Autodesk Fusion 360 part; units mm, degrees
(part 4 of 4)
  spline S3 degree 5 poles (40.8877, 43.7518) (40.9094, 43.7499) (40.9529, 43.7455) (41.018, 43.7374) (41.1043, 43.7233) (41.2113, 43.6998) (41.317, 43.6706) (41.4211, 43.6359) (41.5232, 43.5957) (41.6229, 43.5502) (41.7199, 43.4994) (41.8136, 43.4432) (41.9039, 43.3818) (41.9906, 43.3154) (42.0736, 43.2441) (42.1528, 43.1684) (42.2283, 43.0887) (42.3, 43.0054) (42.3678, 42.9189) (42.4312, 42.8292) (42.4898, 42.7365) (42.5431, 42.641) (42.5907, 42.5425) (42.6323, 42.4415) (42.6679, 42.338) (42.6976, 42.2325) (42.7216, 42.1254) (42.7401, 42.0171) (42.7532, 41.9082) (42.7608, 41.7988) (42.7627, 41.6893) (42.7587, 41.58) (42.7486, 41.4712) (42.7322, 41.3632) (42.7097, 41.2561) (42.6811, 41.1503) (42.6468, 41.0461) (42.6069, 40.9437) (42.5616, 40.8437) (42.511, 40.7464) (42.4551, 40.6523) (42.3941, 40.5617) (42.328, 40.475) (42.257, 40.3921) (42.1815, 40.3132) (42.1021, 40.238) (42.0191, 40.1663) (41.9329, 40.0981) (41.844, 40.0337) (41.7523, 39.9734) (41.6578, 39.9179) (41.5605, 39.8679) (41.4603, 39.8242) (41.3575, 39.787) (41.2523, 39.7567) (41.1453, 39.7331) (41.037, 39.7157) (40.9279, 39.704) (40.8186, 39.6971) (40.7091, 39.6938) (40.5997, 39.693) (40.4904, 39.6936) (40.381, 39.6947) (40.2717, 39.6955) (40.1623, 39.6958) (40.0529, 39.6956) (39.9435, 39.6951) (39.834, 39.6945) (39.7246, 39.6941) (39.6152, 39.694) (39.5058, 39.6941) (39.3964, 39.6944) (39.287, 39.6946) (39.1776, 39.6948) (39.0682, 39.6948) (38.9588, 39.6948) (38.8494, 39.6947) (38.74, 39.6946) (38.6306, 39.6945) (38.5212, 39.6945) (38.4118, 39.6945) (38.3024, 39.6945) (38.193, 39.6946) (38.0836, 39.6946) (37.9742, 39.6946) (37.8648, 39.6946) (37.7554, 39.6946) (37.646, 39.6946) (37.5366, 39.6946) (37.4272, 39.6946) (37.3178, 39.6946) (37.2084, 39.6946) (37.099, 39.6946) (36.9896, 39.6946) (36.8802, 39.6946) (36.7708, 39.6946) (36.6614, 39.6946) (36.552, 39.6946) (36.4425, 39.6946) (36.3331, 39.6946) (36.2237, 39.6946) (36.1143, 39.6946) (36.0049, 39.6946) (35.8955, 39.6946) (35.7861, 39.6946) (35.6767, 39.6946) (35.5673, 39.6946) (35.4579, 39.6946) (35.3485, 39.6945) (35.2391, 39.6945) (35.1297, 39.6945) (35.0203, 39.6945) (34.9109, 39.6946) (34.8015, 39.6946) (34.6922, 39.6947) (34.5828, 39.6947) (34.4734, 39.6947) (34.3639, 39.6946) (34.2544, 39.6944) (34.1449, 39.6943) (34.0355, 39.6942) (33.9262, 39.6943) (33.8169, 39.6946) (33.7077, 39.6949) (33.5984, 39.6952) (33.4891, 39.6952) (33.3796, 39.6949) (33.2699, 39.6945) (33.1601, 39.6949) (33.0503, 39.697) (32.9408, 39.7026) (32.832, 39.7131) (32.7241, 39.7298) (32.6176, 39.7538) (32.5128, 39.785) (32.41, 39.8233) (32.3094, 39.8679) (32.2115, 39.918) (32.1163, 39.9732) (32.0243, 40.033) (31.9357, 40.0972) (31.8507, 40.1659) (31.7695, 40.239) (31.6923, 40.3165) (31.6193, 40.3982) (31.5506, 40.4837) (31.4863, 40.5727) (31.4266, 40.6647) (31.3715, 40.7596) (31.3215, 40.8569) (31.2765, 40.9566) (31.237, 41.0585) (31.203, 41.1625) (31.1748, 41.2682) (31.1527, 41.3755) (31.1366, 41.4839) (31.1266, 41.5931) (31.1229, 41.7026) (31.1253, 41.8121) (31.1336, 41.9212) (31.1477, 42.0297) (31.1675, 42.1374) (31.1927, 42.244) (31.2232, 42.3492) (31.2592, 42.4526) (31.3007, 42.5538) (31.3478, 42.6525) (31.4006, 42.7483) (31.459, 42.8409) (31.5226, 42.93) (31.5911, 43.0155) (31.6642, 43.0974) (31.7412, 43.1754) (31.822, 43.2495) (31.9062, 43.3196) (31.9937, 43.3855) (32.0844, 43.447) (32.1781, 43.5038) (32.2748, 43.5555) (32.3743, 43.6017) (32.4762, 43.6419) (32.5802, 43.6759) (32.686, 43.7035) (32.7933, 43.7249) (32.9016, 43.7405) (33.0106, 43.7511) (33.1201, 43.7577) (33.2297, 43.7613) (33.3393, 43.7627) (33.4487, 43.7627) (33.5581, 43.7621) (33.6674, 43.7612) (33.7767, 43.7605) (33.886, 43.76) (33.9954, 43.7599) (34.1048, 43.76) (34.2142, 43.7603) (34.3237, 43.7606) (34.4331, 43.7608) (34.5426, 43.7609) (34.6519, 43.7608) (34.7613, 43.7607) (34.8707, 43.7606) (34.9801, 43.7605) (35.0895, 43.7605) (35.1989, 43.7605) (35.3083, 43.7605) (35.4177, 43.7606) (35.5271, 43.7606) (35.6365, 43.7606) (35.7459, 43.7606) (35.8553, 43.7606) (35.9647, 43.7606) (36.0741, 43.7606) (36.1835, 43.7606) (36.2929, 43.7606) (36.4023, 43.7606) (36.5117, 43.7606) (36.6211, 43.7606) (36.7305, 43.7606) (36.84, 43.7606) (36.9494, 43.7606) (37.0588, 43.7606) (37.1682, 43.7606) (37.2776, 43.7606) (37.387, 43.7606) (37.4964, 43.7606) (37.6058, 43.7606) (37.7152, 43.7606) (37.8246, 43.7605) (37.934, 43.7605) (38.0434, 43.7605) (38.1528, 43.7606) (38.2622, 43.7606) (38.3716, 43.7607) (38.481, 43.7607) (38.5904, 43.7607) (38.6998, 43.7606) (38.8092, 43.7604) (38.9186, 43.7603) (39.028, 43.7602) (39.1374, 43.7603) (39.2468, 43.7606) (39.3562, 43.7609) (39.4656, 43.7612) (39.5751, 43.7613) (39.6844, 43.7612) (39.7938, 43.7606) (39.9032, 43.7598) (40.0125, 43.7591) (40.1219, 43.7588) (40.2313, 43.7593) (40.3408, 43.7605) (40.4503, 43.7621) (40.5599, 43.7635) (40.6694, 43.7632) (40.7568, 43.7608) (40.8223, 43.7571) (40.8659, 43.7538) (40.8877, 43.7518) knots 0 0 0 0 0 0 0.00392157 0.00784314 0.01176471 0.01568627 0.01960784 0.02352941 0.02745098 0.03137255 0.03529412 0.03921569 0.04313725 0.04705882 0.05098039 0.05490196 0.05882353 0.0627451 0.06666667 0.07058824 0.0745098 0.07843137 0.08235294 0.08627451 0.09019608 0.09411765 0.09803922 0.10196078 0.10588235 0.10980392 0.11372549 0.11764706 0.12156863 0.1254902 0.12941176 0.13333333 0.1372549 0.14117647 0.14509804 0.14901961 0.15294118 0.15686275 0.16078431 0.16470588 0.16862745 0.17254902 0.17647059 0.18039216 0.18431373 0.18823529 0.19215686 0.19607843 0.2 0.20392157 0.20784314 0.21176471 0.21568627 0.21960784 0.22352941 0.22745098 0.23137255 0.23529412 0.23921569 0.24313725 0.24705882 0.25098039 0.25490196 0.25882353 0.2627451 0.26666667 0.27058824 0.2745098 0.27843137 0.28235294 0.28627451 0.29019608 0.29411765 0.29803922 0.30196078 0.30588235 0.30980392 0.31372549 0.31764706 0.32156863 0.3254902 0.32941176 0.33333333 0.3372549 0.34117647 0.34509804 0.34901961 0.35294118 0.35686275 0.36078431 0.36470588 0.36862745 0.37254902 0.37647059 0.38039216 0.38431373 0.38823529 0.39215686 0.39607843 0.4 0.40392157 0.40784314 0.41176471 0.41568627 0.41960784 0.42352941 0.42745098 0.43137255 0.43529412 0.43921569 0.44313725 0.44705882 0.45098039 0.45490196 0.45882353 0.4627451 0.46666667 0.47058824 0.4745098 0.47843137 0.48235294 0.48627451 0.49019608 0.49411765 0.49803922 0.50196078 0.50588235 0.50980392 0.51372549 0.51764706 0.52156863 0.5254902 0.52941176 0.53333333 0.5372549 0.54117647 0.54509804 0.54901961 0.55294118 0.55686275 0.56078431 0.56470588 0.56862745 0.57254902 0.57647059 0.58039216 0.58431373 0.58823529 0.59215686 0.59607843 0.6 0.60392157 0.60784314 0.61176471 0.61568627 0.61960784 0.62352941 0.62745098 0.63137255 0.63529412 0.63921569 0.64313725 0.64705882 0.65098039 0.65490196 0.65882353 0.6627451 0.66666667 0.67058824 0.6745098 0.67843137 0.68235294 0.68627451 0.69019608 0.69411765 0.69803922 0.70196078 0.70588235 0.70980392 0.71372549 0.71764706 0.72156863 0.7254902 0.72941176 0.73333333 0.7372549 0.74117647 0.74509804 0.74901961 0.75294118 0.75686275 0.76078431 0.76470588 0.76862745 0.77254902 0.77647059 0.78039216 0.78431373 0.78823529 0.79215686 0.79607843 0.8 0.80392157 0.80784314 0.81176471 0.81568627 0.81960784 0.82352941 0.82745098 0.83137255 0.83529412 0.83921569 0.84313725 0.84705882 0.85098039 0.85490196 0.85882353 0.8627451 0.86666667 0.87058824 0.8745098 0.87843137 0.88235294 0.88627451 0.89019608 0.89411765 0.89803922 0.90196078 0.90588235 0.90980392 0.91372549 0.91764706 0.92156863 0.9254902 0.92941176 0.93333333 0.9372549 0.94117647 0.94509804 0.94901961 0.95294118 0.95686275 0.96078431 0.96470588 0.96862745 0.97254902 0.97647059 0.98039216 0.98431373 0.98823529 0.99215686 0.99607843 1 1 1 1 1 1
  point P0 (47.9215, 72.9576)
  point P1 (48.4702, 72.8769)
  point P2 (49.0161, 72.7805)
  point P3 (49.5581, 72.6648)
  point P4 (50.0918, 72.5165)
  point P5 (50.6215, 72.3558)
  point P6 (51.1435, 72.171)
  point P7 (51.6562, 71.9628)
  point P8 (52.1629, 71.7382)
  point P9 (52.6554, 71.4852)
  point P10 (53.1393, 71.215)
  point P11 (53.6132, 70.9281)
  point P12 (54.0761, 70.6237)
  point P13 (54.5279, 70.3027)
  point P14 (54.9671, 69.964)
  point P15 (55.3873, 69.6016)
  point P16 (55.7975, 69.2281)
  point P17 (56.1881, 68.834)
  point P18 (56.5593, 68.4216)
  point P19 (56.9182, 67.9986)
  point P20 (57.2575, 67.5599)
  point P21 (57.582, 67.1104)
  point P22 (57.8848, 66.6464)
  point P23 (58.1692, 66.171)
  point P24 (58.4379, 65.6865)
  point P25 (58.6841, 65.1896)
  point P26 (58.9068, 64.683)
  point P27 (59.1142, 64.1696)
  point P28 (59.5316, 63.8586)
  point P29 (60.0421, 63.6449)
  point P30 (60.5476, 63.4178)
  point P31 (61.042, 63.1672)
  point P32 (61.5236, 62.8936)
  point P33 (61.9946, 62.6021)
  point P34 (62.4534, 62.2913)
  point P35 (62.8966, 61.9579)
  point P36 (63.3303, 61.6119)
  point P37 (63.7474, 61.246)
  point P38 (64.1551, 60.8697)
  point P39 (64.5428, 60.4727)
  point P40 (64.9129, 60.0594)
  point P41 (65.2657, 59.6314)
  point P42 (65.6007, 59.1895)
  point P43 (65.9224, 58.738)
  point P44 (66.2228, 58.2724)
  point P45 (66.5057, 57.796)
  point P46 (66.7674, 57.3077)
  point P47 (67.0123, 56.8115)
  point P48 (67.2308, 56.3023)
  point P49 (67.4271, 55.7848)
  point P50 (67.606, 55.2606)
  point P51 (67.7736, 54.7327)
  point P52 (67.9053, 54.1944)
  point P53 (68.0248, 53.6533)
  point P54 (68.112, 53.1057)
  point P55 (68.1767, 52.5549)
  point P56 (68.2351, 52.0033)
  point P57 (68.249, 51.4486)
  point P58 (68.25, 50.8937)
  point P59 (68.2495, 50.3387)
  point P60 (68.2126, 49.7854)
  point P61 (68.1435, 49.235)
  point P62 (68.0572, 48.6872)
  point P63 (67.9523, 48.1428)
  point P64 (67.8163, 47.6059)
  point P65 (67.6733, 47.0707)
  point P66 (67.4992, 46.5447)
  point P67 (67.3027, 46.0271)
  point P68 (67.0815, 45.5197)
  point P69 (66.8456, 45.0184)
  point P70 (66.5847, 44.5296)
  point P71 (66.3047, 44.0517)
  point P72 (66.003, 43.5866)
  point P73 (65.683, 43.1338)
  point P74 (65.3446, 42.6943)
  point P75 (64.9949, 42.2641)
  point P76 (65.0476, 41.7178)
  point P77 (65.1148, 41.1677)
  point P78 (65.1637, 40.615)
  point P79 (65.1808, 40.0604)
  point P80 (65.1782, 39.5055)
  point P81 (65.1586, 38.9509)
  point P82 (65.1109, 38.3981)
  point P83 (65.0454, 37.8476)
  point P84 (64.9561, 37.3006)
  point P85 (64.8392, 36.759)
  point P86 (64.7059, 36.2212)
  point P87 (64.5429, 35.6918)
  point P88 (64.362, 35.1685)
  point P89 (64.1647, 34.6511)
  point P90 (63.9475, 34.1418)
  point P91 (63.7122, 33.6399)
  point P92 (63.4598, 33.1464)
  point P93 (63.1814, 32.6675)
  point P94 (62.8832, 32.2001)
  point P95 (62.5625, 31.7478)
  point P96 (62.2276, 31.3058)
  point P97 (61.8776, 30.8756)
  point P98 (61.5099, 30.4601)
  point P99 (61.1225, 30.0629)
  point P100 (60.7194, 29.6816)
  point P101 (60.3015, 29.3166)
  point P102 (59.869, 28.9693)
  point P103 (59.426, 28.636)
  point P104 (58.966, 28.3265)
  point P105 (58.4964, 28.0324)
  point P106 (58.0156, 27.7575)
  point P107 (57.5265, 27.4992)
  point P108 (57.0237, 27.2687)
  point P109 (56.5128, 27.0555)
  point P110 (55.9932, 26.8631)
  point P111 (55.4664, 26.6917)
  point P112 (54.9312, 26.5488)
  point P113 (54.3934, 26.4161)
  point P114 (53.8492, 26.3097)
  point P115 (53.3013, 26.2235)
  point P116 (52.749, 26.1699)
  point P117 (52.1966, 26.1203)
  point P118 (51.6418, 26.1074)
  point P119 (51.0869, 26.1104)
  point P120 (50.5323, 26.1285)
  point P121 (49.9803, 26.1839)
  point P122 (49.4297, 26.2488)
  point P123 (48.912, 26.1996)
  point P124 (48.4809, 25.8503)
  point P125 (48.0343, 25.5214)
  point P126 (47.5779, 25.2068)
  point P127 (47.1078, 24.9133)
  point P128 (46.6285, 24.636)
  point P129 (46.1351, 24.3838)
  point P130 (45.6315, 24.1538)
  point P131 (45.1199, 23.9423)
  point P132 (44.5994, 23.7539)
  point P133 (44.0704, 23.5904)
  point P134 (43.5373, 23.4403)
  point P135 (42.9951, 23.3256)
  point P136 (42.4494, 23.2296)
  point P137 (41.9007, 23.1492)
  point P138 (41.3496, 23.0854)
  point P139 (40.7955, 23.0575)
  point P140 (40.2406, 23.0536)
  point P141 (39.6857, 23.0563)
  point P142 (39.1314, 23.0801)
  point P143 (38.5804, 23.1453)
  point P144 (38.0317, 23.2253)
  point P145 (37.4859, 23.3214)
  point P146 (36.9434, 23.4345)
  point P147 (36.4092, 23.581)
  point P148 (35.8773, 23.7362)
  point P149 (35.3559, 23.9223)
  point P150 (34.8426, 24.13)
  point P151 (34.3375, 24.3561)
  point P152 (33.846, 24.6098)
  point P153 (33.3596, 24.8745)
  point P154 (32.8857, 25.1617)
  point P155 (32.4233, 25.4674)
  point P156 (31.9694, 25.7858)
  point P157 (31.5305, 26.1248)
  point P158 (31.1077, 26.4841)
  point P159 (30.6997, 26.8601)
  point P160 (30.3078, 27.253)
  point P161 (29.934, 27.663)
  point P162 (29.5741, 28.0853)
  point P163 (29.2332, 28.5228)
  point P164 (28.9115, 28.9744)
  point P165 (28.6046, 29.436)
  point P166 (28.3191, 29.9109)
  point P167 (28.0549, 30.3978)
  point P168 (27.8036, 30.8906)
  point P169 (27.5815, 31.3982)
  point P170 (27.3745, 31.9114)
  point P171 (26.9733, 32.2362)
  point P172 (26.4617, 32.4482)
  point P173 (25.9597, 32.6825)
  point P174 (25.4662, 32.9334)
  point P175 (24.9835, 33.2057)
  point P176 (24.5103, 33.4937)
  point P177 (24.0487, 33.8007)
  point P178 (23.6051, 34.1335)
  point P179 (23.1722, 34.4802)
  point P180 (22.7548, 34.8459)
  point P181 (22.3485, 35.2237)
  point P182 (21.9591, 35.619)
  point P183 (21.5898, 36.0332)
  point P184 (21.2339, 36.4586)
  point P185 (20.8999, 36.9012)
  point P186 (20.5778, 37.3526)
  point P187 (20.2804, 37.8205)
  point P188 (19.9966, 38.2963)
  point P189 (19.7306, 38.7817)
  point P190 (19.4885, 39.279)
  point P191 (19.2698, 39.7879)
  point P192 (19.0752, 40.306)
  point P193 (18.8954, 40.8301)
  point P194 (18.7319, 41.3593)
  point P195 (18.607, 41.8993)
  point P196 (18.4952, 42.442)
  point P197 (18.4017, 42.9883)
  point P198 (18.3273, 43.5376)
  point P199 (18.2664, 44.089)
  point P200 (18.2522, 44.6437)
  point P201 (18.2507, 45.1986)
  point P202 (18.263, 45.7533)
  point P203 (18.3192, 46.3051)
  point P204 (18.3818, 46.8562)
  point P205 (18.4663, 47.4043)
  point P206 (18.5782, 47.9472)
  point P207 (18.7076, 48.4859)
  point P208 (18.8631, 49.0172)
  point P209 (19.0348, 49.5435)
  point P210 (19.2319, 50.0607)
  point P211 (19.4442, 50.572)
  point P212 (19.6738, 51.0764)
  point P213 (19.9353, 51.5652)
  point P214 (20.2124, 52.0448)
  point P215 (20.507, 52.5143)
  point P216 (20.8178, 52.9729)
  point P217 (21.1502, 53.4169)
  point P218 (21.4924, 53.8519)
  point P219 (21.422, 54.3987)
  point P220 (21.3645, 54.9506)
  point P221 (21.3157, 55.503)
  point P222 (21.3041, 56.0578)
  point P223 (21.3057, 56.6127)
  point P224 (21.3199, 57.1674)
  point P225 (21.3719, 57.7197)
  point P226 (21.4294, 58.2715)
  point P227 (21.5206, 58.8185)
  point P228 (21.6429, 59.359)
  point P229 (21.7782, 59.8963)
  point P230 (21.9446, 60.4246)
  point P231 (22.1245, 60.9482)
  point P232 (22.3222, 61.4655)
  point P233 (22.5361, 61.9763)
  point P234 (22.7746, 62.4755)
  point P235 (23.0264, 62.9679)
  point P236 (23.3058, 63.4464)
  point P237 (23.6041, 63.9133)
  point P238 (23.9246, 64.3658)
  point P239 (24.2582, 64.8088)
  point P240 (24.6097, 65.2377)
  point P241 (24.9763, 65.6542)
  point P242 (25.3623, 66.0528)
  point P243 (25.7624, 66.4373)
  point P244 (26.1835, 66.7984)
  point P245 (26.6196, 67.1408)
  point P246 (27.0633, 67.4732)
  point P247 (27.5223, 67.7838)
  point P248 (27.9918, 68.0779)
  point P249 (28.4735, 68.3509)
  point P250 (28.9625, 68.6097)
  point P251 (29.4659, 68.8387)
  point P252 (29.9766, 69.0525)
  point P253 (30.4964, 69.2442)
  point P254 (31.0235, 69.415)
  point P255 (31.5587, 69.5575)
  point P256 (32.0967, 69.6893)
  point P257 (32.6408, 69.7961)
  point P258 (33.1891, 69.8796)
  point P259 (33.7414, 69.9332)
  point P260 (34.2938, 69.9843)
  point P261 (34.8485, 69.9981)
  point P262 (35.4034, 69.9954)
  point P263 (35.9578, 69.9741)
  point P264 (36.51, 69.9199)
  point P265 (37.0599, 69.8501)
  point P266 (37.577, 69.9106)
  point P267 (38.0109, 70.2562)
  point P268 (38.4612, 70.5799)
  point P269 (38.9196, 70.8915)
  point P270 (39.3913, 71.182)
  point P271 (39.8744, 71.4536)
  point P272 (40.3698, 71.7007)
  point P273 (40.8725, 71.9333)
  point P274 (41.3859, 72.1404)
  point P275 (41.9068, 72.3273)
  point P276 (42.4336, 72.4984)
  point P277 (42.968, 72.6441)
  point P278 (43.5077, 72.7697)
  point P279 (44.0531, 72.869)
  point P280 (44.6016, 72.951)
  point P281 (45.1534, 73.0092)
  point P282 (45.7065, 73.049)
  point P283 (46.2614, 73.0553)
  point P284 (46.8163, 73.0505)
  point P285 (47.2756, 68.9919)
  point P286 (47.8251, 68.9156)
  point P287 (48.3701, 68.8132)
  point P288 (48.9103, 68.6871)
  point P289 (49.4398, 68.523)
  point P290 (49.961, 68.3348)
  point P291 (50.4679, 68.1112)
  point P292 (50.9607, 67.8585)
  point P293 (51.4374, 67.5749)
  point P294 (51.8924, 67.2574)
  point P295 (52.3321, 66.9186)
  point P296 (52.756, 66.5601)
  point P297 (53.1568, 66.1755)
  point P298 (53.5396, 65.773)
  point P299 (53.8939, 65.3456)
  point P300 (54.2267, 64.9014)
  point P301 (54.5295, 64.4364)
  point P302 (54.8078, 63.957)
  point P303 (55.0547, 63.4603)
  point P304 (55.2788, 62.9538)
  point P305 (55.4736, 62.4346)
  point P306 (55.6467, 61.908)
  point P307 (55.8439, 61.3916)
  point P308 (56.1684, 60.9439)
  point P309 (56.6144, 60.6169)
  point P310 (57.1298, 60.4154)
  point P311 (57.6624, 60.2612)
  point P312 (58.1825, 60.0688)
  point P313 (58.6887, 59.8441)
  point P314 (59.1863, 59.5983)
  point P315 (59.6702, 59.3281)
  point P316 (60.1341, 59.024)
  point P317 (60.5823, 58.697)
  point P318 (61.0061, 58.3382)
  point P319 (61.4132, 57.9604)
  point P320 (61.7929, 57.5552)
  point P321 (62.1547, 57.1339)
  point P322 (62.4843, 56.6872)
  point P323 (62.7899, 56.2241)
  point P324 (63.0633, 55.7416)
  point P325 (63.3145, 55.2481)
  point P326 (63.535, 54.7393)
  point P327 (63.7263, 54.2194)
  point P328 (63.893, 53.6906)
  point P329 (64.0167, 53.1498)
  point P330 (64.1187, 52.6046)
  point P331 (64.1905, 52.0545)
  point P332 (64.2385, 51.5012)
  point P333 (64.2479, 50.9458)
  point P334 (64.2119, 50.3917)
  point P335 (64.163, 49.8384)
  point P336 (64.0742, 49.2904)
  point P337 (63.9592, 48.7474)
  point P338 (63.8113, 48.213)
  point P339 (63.6315, 47.689)
  point P340 (63.4266, 47.174)
  point P341 (63.1862, 46.6738)
  point P342 (62.9229, 46.1855)
  point P343 (62.6334, 45.7126)
  point P344 (62.3179, 45.256)
  point P345 (61.971, 44.8224)
  point P346 (61.5993, 44.4098)
  point P347 (61.2232, 44.0018)
  point P348 (60.9522, 43.52)
  point P349 (60.8425, 42.9787)
  point P350 (60.8875, 42.4271)
  point P351 (61.0221, 41.8889)
  point P352 (61.1234, 41.3433)
  point P353 (61.2017, 40.7936)
  point P354 (61.2354, 40.2392)
  point P355 (61.2458, 39.6839)
  point P356 (61.2258, 39.1288)
  point P357 (61.1793, 38.5755)
  point P358 (61.0998, 38.0259)
  point P359 (60.9831, 37.4839)
  point P360 (60.8343, 36.9497)
  point P361 (60.6556, 36.4252)
  point P362 (60.4518, 35.9097)
  point P363 (60.2143, 35.4095)
  point P364 (59.9538, 34.9206)
  point P365 (59.664, 34.4475)
  point P366 (59.3438, 33.994)
  point P367 (58.9961, 33.5613)
  point P368 (58.6253, 33.1477)
  point P369 (58.2337, 32.7539)
  point P370 (57.8185, 32.385)
  point P371 (57.3815, 32.0427)
  point P372 (56.926, 31.7261)
  point P373 (56.4574, 31.4291)
  point P374 (55.9708, 31.1644)
  point P375 (55.4714, 30.9256)
  point P376 (54.9558, 30.7226)
  point P377 (54.4322, 30.5405)
  point P378 (53.9014, 30.3806)
  point P379 (53.3589, 30.2652)
  point P380 (52.8111, 30.1768)
  point P381 (52.2588, 30.1183)
  point P382 (51.7037, 30.1)
  point P383 (51.1483, 30.1068)
  point P384 (50.5948, 30.1498)
  point P385 (50.0438, 30.2173)
  point P386 (49.5028, 30.3389)
  point P387 (48.9638, 30.4682)
  point P388 (48.4135, 30.5203)
  point P389 (47.8747, 30.3955)
  point P390 (47.3931, 30.1255)
  point P391 (46.9771, 29.7583)
  point P392 (46.5661, 29.3847)
  point P393 (46.1309, 29.0398)
  point P394 (45.6761, 28.7219)
  point P395 (45.2029, 28.4325)
  point P396 (44.7148, 28.1708)
  point P397 (44.2122, 27.9386)
  point P398 (43.7001, 27.7269)
  point P399 (43.1748, 27.5509)
  point P400 (42.6407, 27.4027)
  point P401 (42.0973, 27.2916)
  point P402 (41.5495, 27.2044)
  point P403 (40.9981, 27.139)
  point P404 (40.443, 27.1206)
  point P405 (39.8876, 27.1277)
  point P406 (39.3343, 27.1716)
  point P407 (38.783, 27.2394)
  point P408 (38.2378, 27.3432)
  point P409 (37.6996, 27.4767)
  point P410 (37.1674, 27.632)
  point P411 (36.6494, 27.8286)
  point P412 (36.142, 28.0524)
  point P413 (35.6483, 28.3038)
  point P414 (35.1673, 28.5802)
  point P415 (34.7012, 28.8813)
  point P416 (34.2581, 29.2156)
  point P417 (33.8327, 29.5725)
  point P418 (33.4311, 29.9562)
  point P419 (33.0505, 30.3607)
  point P420 (32.695, 30.7874)
  point P421 (32.3668, 31.2351)
  point P422 (32.0645, 31.7004)
  point P423 (31.7931, 32.1843)
  point P424 (31.5495, 32.6823)
  point P425 (31.3243, 33.189)
  point P426 (31.1358, 33.7107)
  point P427 (30.9798, 34.2427)
  point P428 (30.7653, 34.7529)
  point P429 (30.4288, 35.1912)
  point P430 (29.9782, 35.512)
  point P431 (29.4576, 35.7009)
  point P432 (28.9264, 35.8592)
  point P433 (28.4095, 36.0585)
  point P434 (27.9043, 36.2863)
  point P435 (27.412, 36.5395)
  point P436 (26.9343, 36.8214)
  point P437 (26.4701, 37.1257)
  point P438 (26.0263, 37.4591)
  point P439 (25.6013, 37.8167)
  point P440 (25.1984, 38.1989)
  point P441 (24.8175, 38.6031)
  point P442 (24.4571, 39.0257)
  point P443 (24.1209, 39.4677)
  point P444 (23.8145, 39.93)
  point P445 (23.5338, 40.4079)
  point P446 (23.2856, 40.9042)
  point P447 (23.0627, 41.4113)
  point P448 (22.8669, 41.93)
  point P449 (22.6955, 42.457)
  point P450 (22.5682, 42.9968)
  point P451 (22.467, 43.5421)
  point P452 (22.4011, 44.0929)
  point P453 (22.3613, 44.647)
  point P454 (22.3529, 45.2023)
  point P455 (22.3871, 45.7566)
  point P456 (22.4331, 46.3102)
  point P457 (22.5214, 46.8583)
  point P458 (22.6458, 47.3989)
  point P459 (22.7924, 47.9338)
  point P460 (22.9732, 48.4578)
  point P461 (23.1844, 48.9703)
  point P462 (23.4249, 49.4701)
  point P463 (23.6958, 49.9537)
  point P464 (23.989, 50.4244)
  point P465 (24.3114, 50.876)
  point P466 (24.6591, 51.3088)
  point P467 (25.0275, 51.7242)
  point P468 (25.405, 52.1312)
  point P469 (25.672, 52.6151)
  point P470 (25.7863, 53.1552)
  point P471 (25.7407, 53.7075)
  point P472 (25.612, 54.2469)
  point P473 (25.5032, 54.7908)
  point P474 (25.436, 55.3419)
  point P475 (25.3846, 55.8946)
  point P476 (25.3773, 56.45)
  point P477 (25.3948, 57.0052)
  point P478 (25.4565, 57.557)
  point P479 (25.5392, 58.1056)
  point P480 (25.6466, 58.6497)
  point P481 (25.7989, 59.1826)
  point P482 (25.9742, 59.7082)
  point P483 (26.1823, 60.2218)
  point P484 (26.4115, 60.7267)
  point P485 (26.6753, 61.2145)
  point P486 (26.9655, 61.6873)
  point P487 (27.285, 62.141)
  point P488 (27.6321, 62.5743)
  point P489 (28.0058, 62.9853)
  point P490 (28.3978, 63.3788)
  point P491 (28.8105, 63.7506)
  point P492 (29.2479, 64.0924)
  point P493 (29.7041, 64.4081)
  point P494 (30.1725, 64.7051)
  point P495 (30.6579, 64.9723)
  point P496 (31.1606, 65.2046)
  point P497 (31.6742, 65.413)
  point P498 (32.198, 65.5931)
  point P499 (32.7297, 65.7486)
  point P500 (33.2716, 65.8671)
  point P501 (33.8194, 65.953)
  point P502 (34.3711, 66.0139)
  point P503 (34.9264, 66.0274)
  point P504 (35.4819, 66.0216)
  point P505 (36.0364, 65.9925)
  point P506 (36.5866, 65.9169)
  point P507 (37.1292, 65.8013)
  point P508 (37.6645, 65.6575)
  point P509 (38.2177, 65.6229)
  point P510 (38.7572, 65.7404)
  point P511 (39.2384, 66.0113)
  point P512 (39.6542, 66.3781)
  point P513 (40.0623, 66.7549)
  point P514 (40.494, 67.1043)
  point P515 (40.9438, 67.4291)
  point P516 (41.4116, 67.7277)
  point P517 (41.8972, 67.9939)
  point P518 (42.3947, 68.2373)
  point P519 (42.9103, 68.4401)
  point P520 (43.4353, 68.6174)
  point P521 (43.9708, 68.7619)
  point P522 (44.5136, 68.8769)
  point P523 (45.063, 68.9573)
  point P524 (45.6168, 68.999)
  point P525 (46.1721, 69.0086)
  point P526 (52.98, 56.1754)
  point P527 (53.4391, 55.8783)
  point P528 (53.7998, 55.468)
  point P529 (54.0329, 54.974)
  point P530 (54.1207, 54.4345)
  point P531 (54.0705, 53.8893)
  point P532 (53.8616, 53.3842)
  point P533 (53.5788, 52.9149)
  point P534 (53.2954, 52.4458)
  point P535 (53.0127, 51.9763)
  point P536 (52.73, 51.5068)
  point P537 (52.4473, 51.0373)
  point P538 (52.1644, 50.5679)
  point P539 (51.8817, 50.0985)
  point P540 (51.599, 49.6289)
  point P541 (51.3166, 49.1593)
  point P542 (51.0341, 48.6898)
  point P543 (50.7517, 48.2202)
  point P544 (50.8514, 47.7392)
  point P545 (51.1336, 47.2696)
  point P546 (51.4165, 46.8003)
  point P547 (51.6995, 46.3312)
  point P548 (51.9826, 45.862)
  point P549 (52.2655, 45.3928)
  point P550 (52.5488, 44.9237)
  point P551 (52.8319, 44.4546)
  point P552 (53.1151, 43.9855)
  point P553 (53.3979, 43.5161)
  point P554 (53.6809, 43.0467)
  point P555 (53.9298, 42.5598)
  point P556 (54.0568, 42.028)
  point P557 (54.0172, 41.4837)
  point P558 (53.855, 40.9619)
  point P559 (53.5562, 40.5042)
  point P560 (53.1429, 40.1458)
  point P561 (52.6502, 39.9107)
  point P562 (52.1117, 39.8179)
  point P563 (51.5702, 39.8857)
  point P564 (51.0625, 40.0844)
  point P565 (50.6289, 40.416)
  point P566 (50.3022, 40.8543)
  point P567 (50.0199, 41.3239)
  point P568 (49.7375, 41.7935)
  point P569 (49.4552, 42.2631)
  point P570 (49.1728, 42.7327)
  point P571 (48.89, 43.2021)
  point P572 (48.6074, 43.6716)
  point P573 (48.3248, 44.1411)
  point P574 (48.0422, 44.6106)
  point P575 (47.7594, 45.08)
  point P576 (47.4766, 45.5495)
  point P577 (47.1937, 46.019)
  point P578 (46.9107, 46.4884)
  point P579 (46.628, 46.9578)
  point P580 (46.3894, 47.4488)
  point P581 (46.2862, 47.9841)
  point P582 (46.3437, 48.5274)
  point P583 (46.5632, 49.0272)
  point P584 (46.8446, 49.4973)
  point P585 (47.1265, 49.9672)
  point P586 (47.4087, 50.437)
  point P587 (47.6909, 50.9067)
  point P588 (47.9728, 51.3765)
  point P589 (48.2547, 51.8464)
  point P590 (48.5367, 52.3162)
  point P591 (48.8189, 52.7857)
  point P592 (49.1011, 53.2554)
  point P593 (49.3833, 53.7251)
  point P594 (49.6654, 54.1949)
  point P595 (49.9478, 54.6644)
  point P596 (50.2298, 55.1341)
  point P597 (50.5216, 55.5979)
  point P598 (50.906, 55.9856)
  point P599 (51.386, 56.2461)
  point P600 (51.9167, 56.3754)
  point P601 (41.42, 43.6347)
  point P602 (41.9017, 43.3816)
  point P603 (42.2977, 43.0062)
  point P604 (42.5883, 42.5439)
  point P605 (42.7384, 42.0197)
  point P606 (42.7474, 41.4749)
  point P607 (42.6071, 40.9481)
  point P608 (42.33, 40.48)
  point P609 (41.937, 40.1027)
  point P610 (41.4656, 39.8282)
  point P611 (40.9353, 39.7059)
  point P612 (40.388, 39.6946)
  point P613 (39.8405, 39.6946)
  point P614 (39.293, 39.6946)
  point P615 (38.7455, 39.6946)
  point P616 (38.198, 39.6946)
  point P617 (37.6505, 39.6946)
  point P618 (37.103, 39.6946)
  point P619 (36.5555, 39.6946)
  point P620 (36.0079, 39.6946)
  point P621 (35.4604, 39.6946)
  point P622 (34.9129, 39.6946)
  point P623 (34.3654, 39.6946)
  point P624 (33.8179, 39.6946)
  point P625 (33.2704, 39.6947)
  point P626 (32.7247, 39.7316)
  point P627 (32.2131, 39.9188)
  point P628 (31.7716, 40.2391)
  point P629 (31.4286, 40.664)
  point P630 (31.2052, 41.1604)
  point P631 (31.1244, 41.6993)
  point P632 (31.193, 42.2397)
  point P633 (31.3994, 42.743)
  point P634 (31.738, 43.1704)
  point P635 (32.1737, 43.4995)
  point P636 (32.6796, 43.7004)
  point P637 (33.2228, 43.7606)
  point P638 (33.7703, 43.7606)
  point P639 (34.3178, 43.7606)
  point P640 (34.8653, 43.7606)
  point P641 (35.4128, 43.7606)
  point P642 (35.9603, 43.7606)
  point P643 (36.5078, 43.7606)
  point P644 (37.0553, 43.7606)
  point P645 (37.6029, 43.7606)
  point P646 (38.1504, 43.7606)
  point P647 (38.6979, 43.7606)
  point P648 (39.2454, 43.7606)
  point P649 (39.7929, 43.7606)
  point P650 (40.3404, 43.7606)
extrude "Codex_Logo_Recess_0_75mm_Bottom" cut sketch "草图24" along normal blind 0.75 bodies 1 in component "01_Integrated_Support_PRINT_BODY"
ref_plane "工作平面5" through (12.125, -1.0675, 2.781) normal (0, -0.358368, 0.93358) x (1, 0, 0) in component "01_Integrated_Support_PRINT_BODY"
ref_plane "工作平面6" through (12.125, -0.311, 0.8101) normal (0, -0.358368, 0.93358) x (1, 0, 0) in component "01_Integrated_Support_PRINT_BODY"
ref_plane "工作平面7" through (12.125, 7.8917, -20.5585) normal (0, -0.358368, 0.93358) x (1, 0, 0) in component "01_Integrated_Support_PRINT_BODY"
ref_plane "工作平面8" through (12.125, 8.6482, -22.5294) normal (0, -0.358368, 0.93358) x (1, 0, 0) in component "01_Integrated_Support_PRINT_BODY"
sketch "草图25" plane through (0, -1.0675, 2.781) normal (0, -0.358368, 0.93358) x (1, 0, 0) in component "01_Integrated_Support_PRINT_BODY"
  circle A0 centre (8.2, 7.7127) radius 1.2
  dimension "d194" = 8.2
  dimension "d195" = 7.7127
  dimension "d196" = 2.4
  measures "d194" horizontal distance of origin A0.centre
  measures "d195" vertical distance of origin A0.centre
  measures "d196" diameter of A0
sketch "草图26" plane through (0, -0.311, 0.8101) normal (0, -0.358368, 0.93358) x (1, 0, 0) in component "01_Integrated_Support_PRINT_BODY"
  circle A0 centre (8.2, 7.7127) radius 2.2
  dimension "d197" = 8.2
  dimension "d198" = 7.7127
  dimension "d199" = 4.4
  measures "d197" horizontal distance of origin A0.centre
  measures "d198" vertical distance of origin A0.centre
  measures "d199" diameter of A0
loft "V05_Vendor_Angle_Bearing_Cone_FrontL" cut profiles "草图25", "草图26" section 1 section 2 bodies 1 in component "01_Integrated_Support_PRINT_BODY"
extrude "V05_Clear_Entry_Tunnel_FrontL" cut sketch "草图26" against normal blind 70 bodies 1 in component "01_Integrated_Support_PRINT_BODY"
sketch "草图27" plane through (0, -1.0675, 2.781) normal (0, -0.358368, 0.93358) x (1, 0, 0) in component "01_Integrated_Support_PRINT_BODY"
  circle A0 centre (78.3, 7.7127) radius 1.2
  dimension "d202" = 78.3
  dimension "d203" = 7.7127
  dimension "d204" = 2.4
  measures "d202" horizontal distance of origin A0.centre
  measures "d203" vertical distance of origin A0.centre
  measures "d204" diameter of A0
sketch "草图28" plane through (0, -0.311, 0.8101) normal (0, -0.358368, 0.93358) x (1, 0, 0) in component "01_Integrated_Support_PRINT_BODY"
  circle A0 centre (78.3, 7.7127) radius 2.2
  dimension "d205" = 78.3
  dimension "d206" = 7.7127
  dimension "d207" = 4.4
  measures "d205" horizontal distance of origin A0.centre
  measures "d206" vertical distance of origin A0.centre
  measures "d207" diameter of A0
loft "V05_Vendor_Angle_Bearing_Cone_FrontR" cut profiles "草图27", "草图28" section 1 section 2 bodies 1 in component "01_Integrated_Support_PRINT_BODY"
extrude "V05_Clear_Entry_Tunnel_FrontR" cut sketch "草图28" against normal blind 70 bodies 1 in component "01_Integrated_Support_PRINT_BODY"
sketch "草图29" plane through (0, 7.8917, -20.5585) normal (0, -0.358368, 0.93358) x (1, 0, 0) in component "01_Integrated_Support_PRINT_BODY"
  circle A0 centre (8.2, 82.0127) radius 1.2
  dimension "d210" = 8.2
  dimension "d211" = 82.0127
  dimension "d212" = 2.4
  measures "d210" horizontal distance of origin A0.centre
  measures "d211" vertical distance of origin A0.centre
  measures "d212" diameter of A0
sketch "草图30" plane through (0, 8.6482, -22.5294) normal (0, -0.358368, 0.93358) x (1, 0, 0) in component "01_Integrated_Support_PRINT_BODY"
  circle A0 centre (8.2, 82.0127) radius 2.2
  dimension "d213" = 8.2
  dimension "d214" = 82.0127
  dimension "d215" = 4.4
  measures "d213" horizontal distance of origin A0.centre
  measures "d214" vertical distance of origin A0.centre
  measures "d215" diameter of A0
loft "V05_Vendor_Angle_Bearing_Cone_RearL" cut profiles "草图29", "草图30" section 1 section 2 bodies 1 in component "01_Integrated_Support_PRINT_BODY"
extrude "V05_Clear_Entry_Tunnel_RearL" cut sketch "草图30" against normal blind 70 bodies 1 in component "01_Integrated_Support_PRINT_BODY"
sketch "草图31" plane through (0, 7.8917, -20.5585) normal (0, -0.358368, 0.93358) x (1, 0, 0) in component "01_Integrated_Support_PRINT_BODY"
  circle A0 centre (78.3, 82.0127) radius 1.2
  dimension "d218" = 78.3
  dimension "d219" = 82.0127
  dimension "d220" = 2.4
  measures "d218" horizontal distance of origin A0.centre
  measures "d219" vertical distance of origin A0.centre
  measures "d220" diameter of A0
sketch "草图32" plane through (0, 8.6482, -22.5294) normal (0, -0.358368, 0.93358) x (1, 0, 0) in component "01_Integrated_Support_PRINT_BODY"
  circle A0 centre (78.3, 82.0127) radius 2.2
  dimension "d221" = 78.3
  dimension "d222" = 82.0127
  dimension "d223" = 4.4
  measures "d221" horizontal distance of origin A0.centre
  measures "d222" vertical distance of origin A0.centre
  measures "d223" diameter of A0
loft "V05_Vendor_Angle_Bearing_Cone_RearR" cut profiles "草图31", "草图32" section 1 section 2 bodies 1 in component "01_Integrated_Support_PRINT_BODY"
extrude "V05_Clear_Entry_Tunnel_RearR" cut sketch "草图32" against normal blind 70 bodies 1 in component "01_Integrated_Support_PRINT_BODY"
ref_plane "工作平面9" through (2.4, 0, 0) normal (1, 0, 0) x (0, 1, 0) in component "01_Integrated_Support_PRINT_BODY"
sketch "草图33" plane through (2.4, 0, 0) normal (1, 0, 0) x (0, 0, -1) in component "01_Integrated_Support_PRINT_BODY"
  ellipse E0 centre (-3.7, 26.3844) end of major axis (-2.4, 26.3844) minor radius 0.1 (-2.4, 26.3844) -> (-3.7, 26.2844) cw
  ellipse E1 centre (-3.7, 24.9844) end of major axis (-2.4, 24.9844) minor radius 0.1 (-2.4, 24.9844) -> (-3.7, 25.0844) ccw
  line L0 (-2.4, 24.9844) -> (-2.4, 26.3844)
  line L1 (-3.7, 26.2844) -> (-8.9, 26.2844)
  line L2 (-8.9, 26.2844) -> (-8.9, 25.0844)
  line L3 (-8.9, 25.0844) -> (-3.7, 25.0844)
extrude "V08_Divider_Join_6p5mm_Height" [suppressed] in component "01_Integrated_Support_PRINT_BODY"
ref_plane "工作平面10" through (8.119, 0, 0) normal (1, 0, 0) x (0, 1, 0) in component "01_Integrated_Support_PRINT_BODY"
sketch "草图35" plane through (8.119, 0, 0) normal (1, 0, 0) x (0, 0, -1) in component "01_Integrated_Support_PRINT_BODY"
  spline S0 degree 5 poles (-2.4, 24.8844) (-2.4, 24.9344) (-2.4, 24.9844) (-2.8333, 25.0344) (-4.3067, 25.0344) (-5.78, 25.0344) (-6.82, 25.0344) (-7.86, 25.0344) (-8.9, 25.0344) knots 0 0 0 0 0 0 0.294118 0.294118 0.294118 1 1 1 1 1 1
  spline S1 degree 5 poles (-2.4, 26.3844) (-2.4, 26.3344) (-2.4, 26.2844) (-2.8333, 26.2344) (-4.3067, 26.2344) (-5.78, 26.2344) (-6.82, 26.2344) (-7.86, 26.2344) (-8.9, 26.2344) knots 0 0 0 0 0 0 0.294118 0.294118 0.294118 1 1 1 1 1 1
  line L0 (-2.4, 24.8844) -> (-2.4, 26.3844)
  line L1 (-8.9, 25.0344) -> (-8.9, 26.2344)
  point P0 (-2.4, 24.9344)
  point P1 (-2.4, 24.9844)
  point P2 (-2.8333, 25.0344)
  point P3 (-4.3067, 25.0344)
  point P4 (-5.78, 25.0344)
  point P5 (-6.82, 25.0344)
  point P6 (-7.86, 25.0344)
  point P7 (-2.4, 26.3344)
  point P8 (-2.4, 26.2844)
  point P9 (-2.8333, 26.2344)
  point P10 (-4.3067, 26.2344)
  point P11 (-5.78, 26.2344)
  point P12 (-6.82, 26.2344)
  point P13 (-7.86, 26.2344)
extrude "V09_Seamless_G2_Divider_7_to_60" add sketch "草图35" along normal blind 43.301 bodies 1 in component "01_Integrated_Support_PRINT_BODY"
component "01_Integrated_Support_PRINT_BODY" placed x (1, 0, 0) y (0, 1, 0) z (0, 0, 1) at (0, 0, 0)
component "02_REFERENCE_ORIGINAL_BOX_NOT_FOR_PRINT" placed x (1, 0, 0) y (0, 1, 0) z (0, 0, 1) at (0, 0, 0)
component "(未保存)" placed x (1, 0, 0) y (0, 1, 0) z (0, 0, 1) at (0, 0, 0) in component "02_REFERENCE_ORIGINAL_BOX_NOT_FOR_PRINT"
hidden bodies 2
equation "boxW = 86.5 mm" comment "Confirmed original outer width"
equation "boxL = 86.5 mm" comment "Confirmed original outer length"
equation "boxT = 14 mm" comment "Confirmed original outer thickness"
equation "tilt = 21 deg" comment "30 deg reduced by 30 percent"
equation "frontZ = 4.5 mm" comment "Provisional clearance for front socket head"
equation "noseSetback = 3 mm" comment "Beveled nose; no vertical low-end wall"
equation "wall = 2.4 mm" comment "Draft printed shell and integrated floor"
equation "originalHeadD = 3.8 mm" comment "Legacy head assumption; no longer used to locate holes in v0.4"
equation "edgeX = 7.2 mm" comment "Measured original outer left/right edge to screw SHANK edge, not screw head"
equation "edgeV = 5.1 mm" comment "Measured original outer top/bottom edge to screw SHANK edge, not screw head"
equation "uLow = edgeX + screwMajorD / 2" comment "Inferred screw axis offset"
equation "uHigh = boxW - uLow" comment "Symmetric right screw axis"
equation "vLow = edgeV + screwMajorD / 2" comment "Inferred front row"
equation "vHigh = boxL - vLow" comment "Symmetric rear row"
equation "projectD = boxL * cos(tilt)" comment "Horizontal projection of mating face"
equation "rearZ = frontZ + boxL * sin(tilt)" comment "High-end height"
equation "entryFront = vLow / cos(tilt) + frontZ * tan(tilt)" comment "Front screw axis at Z=0"
equation "entryRear = vHigh / cos(tilt) + frontZ * tan(tilt)" comment "Rear screw axis at Z=0"
equation "endMargin = entryFront - noseSetback" comment "Equal front and rear bottom edge margins"
equation "baseRear = entryRear + endMargin" comment "Balanced rear extension"
equation "baseL = baseRear - noseSetback" comment "Bottom ground-contact length"
equation "bossD = 6 mm" comment "Local screw reinforcement diameter"
equation "ribT = 2 mm" comment "Radial support web thickness"
equation "clearD = screwMajorD * ( 1 + shaftDiameterAllowance )" comment "Draft M2 clearance hole; calibrate for printer"
equation "headPocketD = 4.4 mm" comment "Draft recess for 3.8 mm socket head"
equation "socketHeadD = 3.8 mm" comment "Vendor image: countersunk head maximum diameter 3.8 mm"
equation "socketHeadH = 1.9 mm" comment "Vendor image: full frustum axial head height 1.9 mm; not a standard-angle assumption"
equation "engagement = boxThreadGap + threadInsertion" comment "Total penetration past original opening/mating plane, including 6.3 mm air gap; NOT just engaged thread"
equation "frontScrewL = 10 mm" comment "Vendor TOTAL length INCLUDING countersunk head"
equation "rearScrewL = 35 mm" comment "Vendor TOTAL length INCLUDING countersunk head"
equation "frontGrip = frontHeadFaceOffset" comment "Legacy datum only: now head OUTER FACE offset, not under-head grip"
equation "rearGrip = rearHeadFaceOffset" comment "Legacy datum only: now head OUTER FACE offset, not under-head grip"
equation "batteryT = 6.5 mm" comment "User maximum thickness; footprint not specified"
equation "cutLength = 70 mm" comment "Through-tool length; not screw length"
equation "d35 = noseSetback"
equation "d36 = baseRear"
equation "d37 = rearZ"
equation "d38 = projectD"
equation "d39 = frontZ"
equation "d40 = boxW"
equation "d42 = boxW"
equation "d44 = wall"
equation "d45 = tilt"
equation "d47 = frontZ * cos(tilt)"
equation "d49 = uLow"
equation "d50 = frontZ * sin(tilt) + vLow"
equation "d51 = bossD"
equation "d52 = -( cutLength )"
equation "d56 = frontZ * sin(tilt) + vLow - ribT / 2"
equation "d57 = uLow"
equation "d58 = ribT"
equation "d59 = -( cutLength )"
equation "d61 = uHigh"
equation "d62 = frontZ * sin(tilt) + vLow"
equation "d63 = bossD"
equation "d64 = -( cutLength )"
equation "d66 = uHigh"
equation "d67 = frontZ * sin(tilt) + vLow - ribT / 2"
equation "d68 = uLow"
equation "d69 = ribT"
equation "d70 = -( cutLength )"
equation "d72 = uLow"
equation "d73 = frontZ * sin(tilt) + vHigh"
equation "d74 = bossD"
equation "d75 = -( cutLength )"
equation "d77 = frontZ * sin(tilt) + vHigh - ribT / 2"
equation "d78 = uLow"
equation "d79 = ribT"
equation "d80 = -( cutLength )"
equation "d82 = uHigh"
equation "d83 = frontZ * sin(tilt) + vHigh"
equation "d84 = bossD"
equation "d85 = -( cutLength )"
equation "d87 = uHigh"
equation "d88 = frontZ * sin(tilt) + vHigh - ribT / 2"
equation "d89 = uLow"
equation "d90 = ribT"
equation "d91 = -( cutLength )"
equation "d93 = -frontGrip"
equation "d95 = -rearGrip"
equation "d97 = uLow"
equation "d98 = frontZ * sin(tilt) + vLow"
equation "d99 = clearD"
equation "d100 = -( cutLength )"
equation "d102 = uLow"
equation "d103 = frontZ * sin(tilt) + vLow"
equation "d104 = headPocketD"
equation "d105 = -( cutLength )"
equation "d107 = uHigh"
equation "d108 = frontZ * sin(tilt) + vLow"
equation "d109 = clearD"
equation "d110 = -( cutLength )"
equation "d112 = uHigh"
equation "d113 = frontZ * sin(tilt) + vLow"
equation "d114 = headPocketD"
equation "d115 = -( cutLength )"
equation "d117 = uLow"
equation "d118 = frontZ * sin(tilt) + vHigh"
equation "d119 = clearD"
equation "d120 = -( cutLength )"
equation "d122 = uLow"
equation "d123 = frontZ * sin(tilt) + vHigh"
equation "d124 = headPocketD"
equation "d125 = -( cutLength )"
equation "d127 = uHigh"
equation "d128 = frontZ * sin(tilt) + vHigh"
equation "d129 = clearD"
equation "d130 = -( cutLength )"
equation "d132 = uHigh"
equation "d133 = frontZ * sin(tilt) + vHigh"
equation "d134 = headPocketD"
equation "d135 = -( cutLength )"
equation "d137 = frontZ * sin(tilt)"
equation "d138 = boxW"
equation "d139 = boxL"
equation "d140 = boxT"
equation "endWebOverlap = 0.3 mm" comment "Positive overlap of end-wall short web with screw boss"
equation "d143 = uLow - ribT / 2"
equation "d144 = frontZ * sin(tilt)"
equation "d145 = ribT"
equation "d146 = vLow - bossD / 2 + endWebOverlap"
equation "d147 = -( cutLength )"
equation "d149 = uHigh - ribT / 2"
equation "d150 = frontZ * sin(tilt)"
equation "d151 = ribT"
equation "d152 = vLow - bossD / 2 + endWebOverlap"
equation "d153 = -( cutLength )"
equation "d155 = uLow - ribT / 2"
equation "d156 = frontZ * sin(tilt) + vHigh + bossD / 2 - endWebOverlap"
equation "d157 = ribT"
equation "d158 = vLow - bossD / 2 + endWebOverlap"
equation "d159 = -( cutLength )"
equation "d161 = uHigh - ribT / 2"
equation "d162 = frontZ * sin(tilt) + vHigh + bossD / 2 - endWebOverlap"
equation "d163 = ribT"
equation "d164 = vLow - bossD / 2 + endWebOverlap"
equation "d165 = -( cutLength )"
equation "logoDepth = 0.75 mm" comment "v0.6: original 0.5 mm recess deepened 50 percent to 0.75 mm; 1.65 mm floor remains"
equation "d168 = logoDepth"
equation "screwMajorD = 2 mm" comment "Nominal M2 screw shank diameter; used for measured edge-to-axis conversion"
equation "shaftDiameterAllowance = 0.2" comment "Diameter allowance relative to M2: 20 percent"
equation "boxThreadGap = 6.3 mm" comment "Measured along screw axis from mating rim/opening plane to top of female seat"
equation "threadInsertion = 1.0 mm" comment "v0.6 user requested nominal tip insertion 1 mm, reducing engagement to increase blind-hole reserve"
equation "assumedSocketDepth = 2 mm" comment "Conservative provisional usable depth; user estimates 2 mm plus"
equation "socketBottomMargin = assumedSocketDepth - threadInsertion" comment "Nominal anti-bottoming reserve; verify actual blind hole"
equation "coneSlope = ( socketHeadD - screwMajorD ) / ( 2 * socketHeadH )" comment "Radius change divided by full vendor head height"
equation "coneIncludedAngle = 2 * atan(coneSlope)" comment "Derived solely from vendor 3.8/2.0/1.9 mm data; ignores image-estimated 98 deg"
equation "frontHeadFaceOffset = frontScrewL - boxThreadGap - threadInsertion" comment "Mating plane to widest OUTER HEAD FACE; total length includes head"
equation "rearHeadFaceOffset = rearScrewL - boxThreadGap - threadInsertion" comment "Mating plane to widest OUTER HEAD FACE; total length includes head"
equation "frontNeckOffset = frontHeadFaceOffset - socketHeadH" comment "Location of nominal frustum-to-shank junction"
equation "rearNeckOffset = rearHeadFaceOffset - socketHeadH" comment "Location of nominal frustum-to-shank junction"
equation "frontConeThroat = frontHeadFaceOffset - ( socketHeadD - clearD ) / ( 2 * coneSlope )" comment "Position where bearing cone intersects 2.4 mm clearance bore"
equation "rearConeThroat = rearHeadFaceOffset - ( socketHeadD - clearD ) / ( 2 * coneSlope )" comment "Position where bearing cone intersects 2.4 mm clearance bore"
equation "frontConeEntry = frontHeadFaceOffset + ( headPocketD - socketHeadD ) / ( 2 * coneSlope )" comment "Extend matching cone to 4.4 mm entry before cylindrical access"
equation "rearConeEntry = rearHeadFaceOffset + ( headPocketD - socketHeadD ) / ( 2 * coneSlope )" comment "Extend matching cone to 4.4 mm entry before cylindrical access"
equation "d186 = -frontConeThroat"
equation "d188 = -frontConeEntry"
equation "d190 = -rearConeThroat"
equation "d192 = -rearConeEntry"
equation "d194 = uLow"
equation "d195 = frontZ * sin(tilt) + vLow"
equation "d196 = clearD"
equation "d197 = uLow"
equation "d198 = frontZ * sin(tilt) + vLow"
equation "d199 = headPocketD"
equation "d200 = -( cutLength )"
equation "d202 = uHigh"
equation "d203 = frontZ * sin(tilt) + vLow"
equation "d204 = clearD"
equation "d205 = uHigh"
equation "d206 = frontZ * sin(tilt) + vLow"
equation "d207 = headPocketD"
equation "d208 = -( cutLength )"
equation "d210 = uLow"
equation "d211 = frontZ * sin(tilt) + vHigh"
equation "d212 = clearD"
equation "d213 = uLow"
equation "d214 = frontZ * sin(tilt) + vHigh"
equation "d215 = headPocketD"
equation "d216 = -( cutLength )"
equation "d218 = uHigh"
equation "d219 = frontZ * sin(tilt) + vHigh"
equation "d220 = clearD"
equation "d221 = uHigh"
equation "d222 = frontZ * sin(tilt) + vHigh"
equation "d223 = headPocketD"
equation "d224 = -( cutLength )"
equation "dividerHeight = 6.5 mm" comment "Design record for fixed exact cross-section; edit sketch to change"
equation "dividerThickness = 1.2 mm" comment "Straight wall thickness; fixed exact cross-section"
equation "dividerFarEnvelopeGap = 22.1 mm" comment "Measured along inner floor from low-end inner wall to farthest foot edge"
equation "dividerRootHeight = 1.3 mm" comment "Lower 20 percent; fixed elliptical arcs"
equation "dividerRootSpreadEach = 0.1 mm" comment "Each side root spread; total 0.2 mm maximum"
equation "dividerSpan = 81.7 mm" comment "Driven extrusion span between original sidewalls"
equation "d234 = dividerSpan"
equation "dividerOriginalSpan = 81.7 mm" comment "v0.8 full divider span between sidewalls"
equation "dividerStartFraction = 0.07" comment "Keep from 7 percent of original wall"
equation "dividerEndFraction = 0.60" comment "Keep to 60 percent of original wall"
equation "dividerV09StartX = wall + dividerOriginalSpan * dividerStartFraction" comment "Start from original X-low wall end"
equation "dividerV09Span = dividerOriginalSpan * ( dividerEndFraction - dividerStartFraction )" comment "Retained wall length"
equation "dividerV09RootSpreadEach = 0.15 mm" comment "Fixed cross section record; 50 percent greater than v0.8"
equation "dividerV09RootHeight = 1.3 mm" comment "Lower 20 percent; fixed cross section record"
equation "d243 = dividerV09StartX"
equation "d247 = dividerV09Span"
named bodies: "Support_v0.9_Partial_G2_Divider_Codex", "REFERENCE_ENVELOPE_DO_NOT_PRINT", "ORIGINAL_BOX_ENVELOPE_DO_NOT_PRINT"
